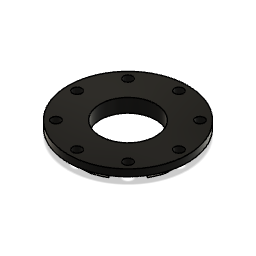
vertical transfer rod handle v6 (Autodesk Fusion 360 design; units mm, degrees)
Autodesk Fusion 360 part; units mm, degrees
note: some values were not read from the file. Set by a fixed rule: the direction of a hole.
sketch "Sketch1" plane through (0, 0, 0) normal (0, 1, 0) x (1, 0, 0)
  circle A0 centre (0, 0) radius 34.5
  circle A1 centre (0, 0) radius 20.5
  circle A2 centre (0, 0) radius 37.5 construction
  circle A3 centre (-37.5, 0) radius 3
  circle A4 centre (0, 0) radius 44
  line L0 (-42.8486, 10) -> (-37.5, 10)
  arc A5 (-37.5, -10) -> (-37.5, 10) centre (-37.5, 0) ccw
  line L1 (-37.5, -10) -> (-42.8486, -10)
  circle A6 centre (0, 0) radius 50
  dimension "d1" = 69
  dimension "d2" = 41
  dimension "d3" = 6
  dimension "d6" = 88
  dimension "d7" = 20
  dimension "d26" = 100
  constraint coincident A0.centre A1.centre
  constraint concentric A0 A1
  constraint concentric A1 A2
  constraint coincident A2 A3.centre
  constraint horizontal A0.centre A3.centre
  constraint tangent A0 A3
  constraint concentric A1 A4
  constraint coincident A4 L0.start
  constraint horizontal L0
  constraint tangent L0 A5
  constraint coincident A4 L1.end
  constraint tangent A5 L1
  constraint parallel L0 L1
  constraint coincident A3.centre A5.centre
  constraint concentric A0 A6
  measures "d1" diameter of A0
  measures "d2" diameter of A1
  measures "d3" diameter of A3
  measures "d6" diameter of A4
  measures "d7" distance of L0 L1
  measures "d26" diameter of A6
extrude "Extrude1" add sketch "Sketch1" along normal blind 10 contours A0 A5 | A0 A4 L0 A5 L1 | A0 A5 | A3 | A0 A4 L0 A5 L1 makes body 1
hole "Hole1" at (-37.5, 0, 0) direction (0, 1, 0) diameter 6.6 end through all bodies 1
chamfer "Chamfer1" distance 5 angle 45 1 edges at (-41.0224, 0, 15.9111) on bodies 1
extrude "Extrude2" cut sketch "Sketch1" along normal blind 5 contours A0 A5 | A3 | A0 A4 L0 A5 L1 picked at (-32.255, 1.9522) picked at (-39.9357, 5.9419) bodies 1
pattern_circular "C-Pattern1" count 8 over 360 about axis through (0, 1.75, 0) along (0, 1, 0) of "Hole1", "Extrude2"
extrude "Extrude3" add sketch "Sketch1" along normal blind 60 separate body contours A0 A5 | A0 A4 L0 A5 L1 | A0 A5 | A3 | A0 A4 L0 A5 L1 | A6 makes body 2
hole "Hole2" at (-37.5, 0, 0) direction (0, 1, 0) diameter 6.6 depth 65 tip angle 118 bodies 2
pattern_circular "C-Pattern2" count 8 over 360 about axis through (0, 1.75, 0) along (0, 1, 0) of "Hole2"
extrude "Extrude4" cut sketch "Sketch1" along normal blind 45 contours A0 A4 L0 A5 L1 | A3 | A0 A4 L0 A5 L1 | A6 bodies 2
chamfer "Chamfer3" distance 1 angle 45 2 edges at (-46.6164, 45, 18.0808) (-46.6164, 60, 18.0808) on bodies 2
copy_body "Body->Comp1" bodies 1 removing the originals makes body 3 in component "bottom"
copy_body "Body->Comp2" bodies 2 removing the originals makes body 4 in component "top"
component "bottom" placed x (1, 0, 0) y (0, 1, 0) z (0, 0, 1) at (0, 0, 0)
component "top" placed x (1, 0, 0) y (0, 1, 0) z (0, 0, 1) at (0, 0, 0)
equation "d1 = ( 34.5 * 2 ) * 1 mm"
named bodies: "bottom", "top"
